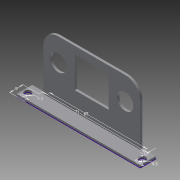
# Autodesk Inventor part: MotorBar
Saved by Autodesk Inventor 2014 SP1 (Build 180222100, 222)
## iProperties
Created: 2015-03-30
Part Number: MotorBar
Material: Generic
Document SubType Name: Modeling
Designer: Erin
Density: 1 g/cm^3
Appearance: Default
Author: Erin
Autodesk Inventor part; units mm, degrees
ref_plane "YZ Plane" through (0, 0, 0) normal (1, 0, 0) x (0, 1, 0)
ref_plane "XZ Plane" through (0, 0, 0) normal (0, 1, 0) x (-1, 0, 0)
ref_plane "XY Plane" through (0, 0, 0) normal (0, 0, 1) x (1, 0, 0)
sketch "Sketch1" plane through (0, 0, 0) normal (0, 0, 1) x (1, 0, 0)
  line L0 (-35.5, 4.5) -> (35.5, 4.5)
  line L1 (35.5, 4.5) -> (35.5, -4.5)
  line L2 (35.5, -4.5) -> (-35.5, -4.5)
  line L3 (-35.5, -4.5) -> (-35.5, 4.5)
  line L4 (-35.5, 4.5) -> (-41.5, 4.5)
  line L5 (-41.5, 4.5) -> (-41.5, -4.5)
  line L6 (-41.5, -4.5) -> (-35.5, -4.5)
  line L7 (-35.5, -4.5) -> (-35.5, 4.5)
  line L8 (35.5, 4.5) -> (41.5, 4.5)
  line L9 (41.5, 4.5) -> (41.5, -4.5)
  line L10 (41.5, -4.5) -> (35.5, -4.5)
  line L11 (35.5, -4.5) -> (35.5, 4.5)
  line L12 (-41.5, 0) -> (41.5, 0) construction
  circle A0 centre (-38.5, 0) radius 2.25
  circle A1 centre (38.5, 0) radius 2.25
  line L13 (0, 4.5) -> (0, -4.5) construction
  line L14 (-32.5, 4.5) -> (32.5, 4.5)
  line L15 (32.5, 4.5) -> (32.5, 6)
  line L16 (32.5, 6) -> (-32.5, 6)
  line L17 (-32.5, 6) -> (-32.5, 4.5)
  line L18 (-32.5, 6) -> (-41.5, 6)
  line L19 (-41.5, 6) -> (-41.5, 4.5)
  line L20 (-41.5, 4.5) -> (-32.5, 4.5)
  line L21 (-32.5, 4.5) -> (-32.5, 6)
  line L22 (32.5, 6) -> (41.5, 6)
  line L23 (41.5, 6) -> (41.5, 4.5)
  line L24 (41.5, 4.5) -> (32.5, 4.5)
  line L25 (32.5, 4.5) -> (32.5, 6)
  point P0 (0, 0)
  point P1 (0, 0)
  point P2 (0, 7)
  point P3 (0, 0)
  point P4 (0, 6)
  dimension "d0" = 9
  dimension "d1" = 71
  dimension "d2" = 4.5
  dimension "d3" = 4.5
  dimension "d4" = 3
  dimension "d5" = 3
  dimension "d6" = 3
  dimension "d7" = 3
  dimension "d12" = 65
  dimension "d13" = 1.5
  constraints: 52 end point, 12 parallel, 7 horizontal, 7 midpoint, 6 perpendicular, 3 point on line, 2 centre point, 2 vertical alignment, 1 coincident, 1 collinear
  measures "d0" distance of L2.end L0.start
  measures "d1" distance of L0.start L0.end
  measures "d2" diameter of A0
  measures "d3" diameter of A1
  measures "d4" distance from line of A1.centre L9
  measures "d5" distance from line of A1.centre L1
  measures "d6" distance from line of A0.centre L5
  measures "d7" distance from line of A0.centre L3
  measures "d12" distance of L15.end L16.end
  measures "d13" distance of L14.end L15.end
extrude "Extrusion1" add sketch "Sketch1" along normal blind 1.5
extrude "Extrusion2" add sketch "Sketch1" along normal blind 40 contours L17 L16 L15 L0
sketch "Sketch2" plane through (-41.5, 4.5, 1.5) normal (0, -1, 0) x (1, 0, 0)
  line L0 (74, 0) -> (74, 38.5) projected
  line L1 (9, 38.5) -> (74, 38.5) projected
  line L2 (9, 0) -> (9, 38.5) projected
  circle A0 centre (19, 23.1) radius 5.5
  circle A1 centre (64, 23.1) radius 5.5
  line L3 (41.5, 38.5) -> (41.5, -1.5) construction
  line L4 (30.1, 33.5) -> (52.9, 33.5)
  line L5 (52.9, 33.5) -> (52.9, 12.7)
  line L6 (52.9, 12.7) -> (30.1, 12.7)
  line L7 (30.1, 12.7) -> (30.1, 33.5)
  line L8 (30.1, 23.1) -> (52.9, 23.1) construction
  point P0 (41.5, 33.5)
  dimension "d16" = 11
  dimension "d17" = 11
  dimension "d19" = 10
  dimension "d21" = 10
  dimension "d22" = 5
  dimension "d23" = 22.8
  dimension "d24" = 20.8
  constraints: 12 end point, 5 midpoint, 3 parallel, 2 centre point, 2 point on line, 1 horizontal, 1 perpendicular, 1 vertical alignment
  measures "d16" diameter of A0
  measures "d17" diameter of A1
  measures "d19" distance from line of A0.centre L2
  measures "d21" distance from line of A1.centre L0
  measures "d22" distance between parallel lines of L4 L1
  measures "d23" distance of L4.start L4.end
  measures "d24" distance of L4.end L5.end
extrude "Extrusion3" cut sketch "Sketch2" against normal blind 10
fillet "Fillet1" radius 10 2 edges at (-32.5, 5.25, 40) (32.5, 5.25, 40)
body "Solid1"
